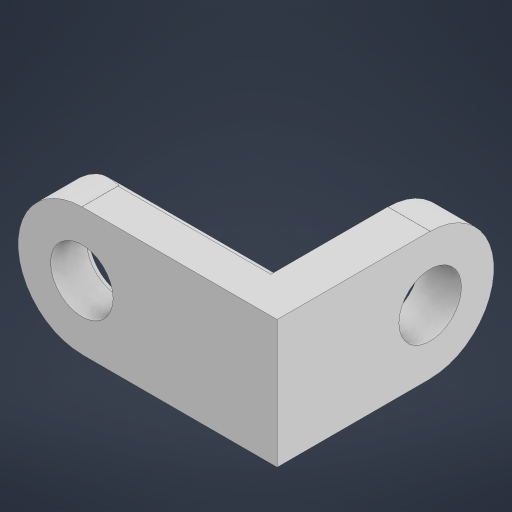
# Autodesk Inventor part: 90joint
Saved by Autodesk Inventor 2023 (Build 270158000, 158)
## iProperties
Created: 2022-04-11
Part Number: 90joint
Material: Generic
Document SubType Name: Modeling
Designer: Vlasciar
Density: 1 g/cm^3
Appearance: Default
Author: Vlasciar
Autodesk Inventor part; units mm, degrees
ref_plane "YZ Plane" through (0, 0, 0) normal (1, 0, 0) x (0, 1, 0)
ref_plane "XZ Plane" through (0, 0, 0) normal (0, 1, 0) x (-1, 0, 0)
ref_plane "XY Plane" through (0, 0, 0) normal (0, 0, 1) x (1, 0, 0)
sketch "Sketch2" plane through (124.0011, 71.4979, 0) normal (0, 0, -1) x (-1, 0, 0)
  line L0 (-1.4859, 28.2151) -> (-1.4859, -1.5861)
  line L1 (-1.4859, -1.5861) -> (34.6281, -1.5861)
  line L2 (34.6281, 28.6132) -> (-1.4859, 28.6132)
  line L3 (-1.4859, 28.6132) -> (-1.4859, 28.2151)
  arc A0 (34.6281, -1.5523) -> (34.6281, 28.5794) centre (34.6281, 13.5135) ccw
  line L4 (34.6281, -1.5861) -> (34.6281, -1.5523)
  line L5 (34.6281, 28.5794) -> (34.6281, 28.6132)
  circle A1 centre (34.6281, 13.5135) radius 7.3816
  point P0 (124.0011, -71.4979)
  constraints: 12 end point, 6 perpendicular, 2 centre point, 2 point on circle, 1 coincident, 1 point on line, 1 vertical
extrude "Extrusion1" add sketch "Sketch2" against normal blind 10
fillet "Fillet1" radius 1.5 3 edges at (107.43, 100.111, 0) (107.43, 69.9118, 0) (125.487, 84.8124, 0)
fillet "Fillet2" radius 1.5 1 edges at (96.7547, 85.0114, 0)
pattern_circular "Circular Pattern1" count 2 over 270 about axis through (125.487, 69.9118, 10) along (0, 1, 0) of "Extrusion1"
body "Solid1"
